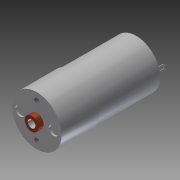
# Autodesk Inventor part: Motor Body
Saved by Autodesk Inventor 2014 (Build 180170000, 170)
## iProperties
Created: 2014-02-03
Part Number: Motor Body
Material: Generic
Document SubType Name: Modeling
Designer: Spooner
Density: 1 g/cm^3
Appearance: Steel
Author: Spooner
Autodesk Inventor part; units mm, degrees
ref_plane "YZ Plane" through (0, 0, 0) normal (1, 0, 0) x (0, 1, 0)
ref_plane "XZ Plane" through (0, 0, 0) normal (0, 1, 0) x (-1, 0, 0)
ref_plane "XY Plane" through (0, 0, 0) normal (0, 0, 1) x (1, 0, 0)
sketch "Sketch1" plane through (0, 0, 0) normal (0, 0, 1) x (1, 0, 0)
  circle A0 centre (0, 0) radius 12.2936
  dimension "d0" = 24.5872
  constraints: 1 centre point, 1 coincident
  measures "d0" diameter of A0
extrude "Extrusion1" add sketch "Sketch1" along normal blind 18.796
sketch "Sketch2" plane through (0, 0, 18.796) normal (0, 0, 1) x (1, 0, 0)
  circle A0 centre (0, 0) radius 12.2936 projected
  circle A1 centre (0, 0) radius 3.4036
  circle A2 centre (0, 0) radius 1.905
  dimension "d3" = 6.8072
  dimension "d6" = 3.81
  constraints: 2 centre point, 2 coincident
  measures "d3" diameter of A1
  measures "d6" diameter of A2
extrude "Extrusion3" add sketch "Sketch2" along normal blind 2.6162 contours A1
sketch "Sketch3" plane through (0, 0, 18.796) normal (0, 0, 1) x (1, 0, 0)
  circle A0 centre (0, 0) radius 12.2936 projected
  point P0 (0, 8.5725)
  point P1 (0, -8.5725)
  dimension "d9" = 17.145
  dimension "d10" = 8.5725
  constraints: 2 vertical alignment
  measures "d9" distance of point (0, -8.572) point (0, 8.572)
  measures "d10" distance of point (0, -8.572) A0.centre
hole "Hole1" at (0, 8.5725, 18.796) at (0, -8.5725, 18.796) direction (0, 0, -1) diameter 2.4638 depth 2.794 tip angle 118
sketch "Sketch4" plane through (0, 0, 0) normal (0, 0, -1) x (-1, 0, 0)
  circle A0 centre (0, 0) radius 12.2936 projected
  circle A1 centre (0, 0) radius 11.8618
  dimension "d18" = 23.7236
  constraints: 1 centre point, 1 coincident
  measures "d18" diameter of A1
extrude "Extrusion4" add sketch "Sketch4" along normal blind 30.5816 contours A1
sketch "Sketch5" plane through (0, 0, -30.5816) normal (0, 0, -1) x (-1, 0, 0)
  circle A0 centre (0, 0) radius 11.8618 projected
  circle A1 centre (0, 0) radius 4.1148
  dimension "d21" = 8.2296
  constraints: 1 centre point, 1 coincident
  measures "d21" diameter of A1
extrude "Extrusion5" add sketch "Sketch5" along normal blind 1.905 contours A1
sketch "Sketch6" plane through (0, 0, -32.4866) normal (0, 0, -1) x (-1, 0, 0)
  circle A0 centre (0, 0) radius 4.1148 projected
  line L0 (-1.9805, -3.6068) -> (1.9805, -3.6068)
  dimension "d24" = 3.6068
  dimension "d25" = 8.2296
  constraints: 2 end point, 2 point on circle, 1 horizontal
  measures "d24" distance from line of L0 A0.centre
  measures "d25" diameter of A0
extrude "Extrusion6" cut sketch "Sketch6" against normal up to surface (1.905 mm away) contours L0 A0 picked at (-0.407, -3.7143)
sketch "Sketch7" plane through (0, 0, -32.4866) normal (0, 0, -1) x (-1, 0, 0)
  arc A0 (1.9805, -3.6068) -> (-1.9805, -3.6068) centre (0, 0) ccw projected
  circle A1 centre (0, 0) radius 0.9906
  dimension "d28" = 1.9812
  constraints: 1 centre point, 1 coincident
  measures "d28" diameter of A1
extrude "Extrusion7" add sketch "Sketch7" along normal blind 0.889
sketch "Sketch8" plane through (0, 0, -30.5816) normal (0, 0, -1) x (-1, 0, 0)
  arc A0 (1.9805, -3.6068) -> (-1.9805, -3.6068) centre (0, 0) ccw projected
  line L0 (-8.6614, 1.5113) -> (-8.4328, 1.5113)
  line L1 (-8.4328, 1.5113) -> (-8.4328, -1.5113)
  line L2 (-8.4328, -1.5113) -> (-8.6614, -1.5113)
  line L3 (-8.6614, -1.5113) -> (-8.6614, 1.5113)
  line L4 (8.4328, 1.5113) -> (8.6614, 1.5113)
  line L5 (8.6614, 1.5113) -> (8.6614, -1.5113)
  line L6 (8.6614, -1.5113) -> (8.4328, -1.5113)
  line L7 (8.4328, -1.5113) -> (8.4328, 1.5113)
  point P0 (-8.4328, 0)
  point P1 (8.4328, 0)
  dimension "d31" = 0.2286
  dimension "d32" = 16.8656
  dimension "d33" = 3.0226
  dimension "d34" = 8.4328
  constraints: 16 end point, 4 horizontal alignment, 4 parallel, 2 horizontal, 2 midpoint, 2 perpendicular, 1 collinear
  measures "d31" distance of L0.start L0.end
  measures "d32" distance between parallel lines of L7 L1
  measures "d33" distance of L4.end L5.end
  measures "d34" distance of point (-8.433, 0) A0.centre
extrude "Extrusion8" add sketch "Sketch8" along normal blind 6.096
sketch "Sketch9" plane through (8.6614, -1.5113, -30.5816) normal (1, 0, 0) x (0, 0, -1)
  line L0 (0, 0) -> (0, 3.0226) projected
  line L1 (0, 0) -> (6.096, 0) projected
  line L2 (6.096, 3.0226) -> (6.096, 0) projected
  line L3 (0, 3.0226) -> (6.096, 3.0226) projected
  arc A0 (4.7498, 0) -> (4.7498, 3.0226) centre (4.5746, 1.5113) ccw
  point P0 (-30.5816, 1.5113)
  dimension "d37" = 1.3462
  constraints: 2 point on circle, 2 point on line, 1 centre point, 1 tangent, 1 vertical alignment
  measures "d37" distance of L2.start A0.end
extrude "Extrusion9" cut sketch "Sketch9" against normal through all contours A0 L2 L1 | L3 L2 A0
sketch "Sketch10" plane through (8.6614, -1.5113, -30.5816) normal (1, 0, 0) x (0, 0, -1)
  arc A0 (4.7498, 0) -> (4.7498, 3.0226) centre (4.5746, 1.5113) ccw projected
  line L0 (0, 0) -> (4.7498, 0) projected
  arc A1 (4.7747, 0.9652) -> (4.7747, 2.0574) centre (4.5746, 1.5113) ccw
  line L1 (3.6073, 0.9652) -> (4.7747, 0.9652)
  line L2 (3.6073, 2.0574) -> (4.7747, 2.0574)
  arc A2 (3.6073, 2.0574) -> (3.6073, 0.9652) centre (3.8074, 1.5113) ccw
  point P0 (-30.5816, 1.5113)
  dimension "d41" = 0.9398
  dimension "d42" = 0.5816
  dimension "d45" = 0.9652
  dimension "d46" = 0.5816
  dimension "d47" = 1.9304
  constraints: 4 end point, 4 point on circle, 2 centre point, 2 vertical alignment, 1 concentric, 1 horizontal, 1 parallel
  measures "d41" radial gap between concentric circles of A0 A1
  measures "d42" radius of A1
  measures "d45" distance between parallel lines of L0 L1
  measures "d46" radius of A2
extrude "Extrusion10" cut sketch "Sketch10" against normal through all
sketch "Sketch11" plane through (0, 0, 18.796) normal (0, 0, 1) x (1, 0, 0)
  circle A0 centre (0, 0) radius 12.2936 projected
  circle A1 centre (-8.3693, 0) radius 2.3622
  circle A2 centre (8.3693, 0) radius 2.3622
  dimension "d50" = 4.7244
  dimension "d51" = 12.0142
  dimension "d53" = 16.7386
  dimension "d54" = 8.3693
  constraints: 2 centre point, 1 equal radius
  measures "d50" diameter of A1
  measures "d53" distance of A1.centre A2.centre
  measures "d54" distance of A2.centre A0.centre
extrude "Extrusion11" cut sketch "Sketch11" against normal blind 0.8636 contours A1 | A2
equation "\"d10\" = 0.5 * d9"
equation "\"d34\" = 0.5 * d32"
equation "\"d46\" = d42"
equation "\"d54\" = 0.5 * d53"
body "Solid1"
